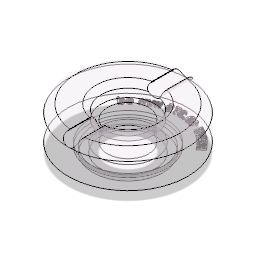
MaxWell_Well_Adapter__Latest_v3 (Autodesk Fusion 360 design; units mm, degrees)
Autodesk Fusion 360 part; units mm, degrees
note: some values were not read from the file. Set by a fixed rule: which face or edge a step refers to.
sketch "Sketch1" plane through (0, 0, 0) normal (0, 1, 0) x (1, 0, 0)
  circle A0 centre (0, 0) radius 16.5
  circle A1 centre (0, 0) radius 5.692
  circle A2 centre (0, 0) radius 7.367
  dimension "d2" = 33
  dimension "d7" = 11.384
  dimension "d21" = 14.734
  constraint coincident A0.centre A1.centre
  constraint concentric A0 A2
  measures "d2" diameter of A0
  measures "d7" diameter of A1
  measures "d21" diameter of A2
extrude "Extrude1" add sketch "Sketch1" along normal blind 9 contours A0
sketch "Sketch2" plane through (0, 0, 0) normal (1, 0, 0) x (0, 0, -1)
  line L0 (16.5, 9) -> (-16.5, 9)
  line L1 (16.5, 0) -> (-16.5, 0)
sketch "Sketch3" plane through (0, 9, 0) normal (0, 1, 0) x (-1, 0, 0)
  circle A0 centre (0, 0) radius 16.5
  line L0 (0, -16.5) -> (0, 16.5)
  line L1 (0, -16.5) -> (0, 16.5)
  line L2 (0, 16.5) -> (-2, 16.5)
  line L3 (0, -16.5) -> (-2, -16.5)
  line L4 (-2, -16.5) -> (-2, 16.5)
  line L5 (-2, 16.5) -> (0, 16.5)
  line L6 (0, 16.5) -> (0, -16.5)
  circle A1 centre (0, 0) radius 7.367
  dimension "d8" = 2
  constraint coincident L0.start L1.start
  constraint coincident L0.end L1.end
  constraint perpendicular L1 L2
  constraint horizontal L3
  constraint vertical L4
  constraint horizontal L5
  constraint vertical L6
  measures "d8" distance of L0.end L2.end
extrude "Extrude3" add sketch "Sketch1" along normal blind 5.95 contours A2
revolve "Revolve1" cut sketch "Sketch3" angle 360 about axis through (0, 9, 16.5) along (0, 0, -1) contours A0 L0 L1 L4 L6 A1 | A0 L2 L4 L5 | A0 L3 L4 | A0 L0 L1 L4 L6 A1 | L0 L1 L4 L6 A1
extrude "Extrude2" add 2 faces at (-4.3141, 9, -12.7105) (4.3141, 9, -12.7105) along direction (0, 1, 0) blind 0.2
fillet "Fillet2" radius 2.2 2 edges at (-16.5, 9.2, 0) (16.5, 9.2, 0)
fillet "Fillet3" radius 1.5 2 edges at (7.367, 9.2, 0) (-7.367, 9.2, 0)
sketch "Sketch5" plane through (0, 0, 0) normal (0, -1, 0) x (1, 0, 0)
  circle A0 centre (0, 0) radius 5.692
  circle A1 centre (0, 0) radius 16.5
  circle A2 centre (0, 0) radius 10.6875
  circle A3 centre (0, 0) radius 9.6875
  circle A4 centre (0, 0) radius 7.6875
  dimension "d29" = 21.375
  dimension "d30" = 19.375
  dimension "d32" = -2
  constraint concentric A0 A2
  constraint concentric A2 A3
  measures "d29" diameter of A2
  measures "d30" diameter of A3
extrude "Extrude5" add sketch "Sketch5" along normal blind 1 contours A2
extrude "Extrude6" add sketch "Sketch5" along normal blind 2.5 contours A3
sketch "Sketch4" plane through (0, 0, 0) normal (0, -1, 0) x (1, 0, 0)
  circle A0 centre (0, 0) radius 16.5
  arc A1 (-16.5, 0) -> (16.5, 0) centre (0, 0) ccw
  arc A2 (-15.5, 0) -> (15.5, 0) centre (0, 0) ccw
  circle A3 centre (0, 0) radius 10.6875
  dimension "d16" = -1
  dimension "d17" = 2
  text T0 "REV7 19.375 mm od" font "Arial" height 2 bold align centre spacing 1.1 along the path A2 letters at x, y, angle (12.9192, -9.5421, -130.0508) (11.4577, -11.2485, -137.7989) (9.8996, -12.6414, -145.2645) (8.1733, -13.8109, -152.1577) (6.6105, -14.6079, -157.0388) (5.7132, -14.9967, -161.9199) (4.0281, -15.5344, -168.2383) (2.3057, -15.8674, -173.1194) (1.3358, -15.9925, -178.0005) (-0.4324, -16.0423, 175.6812) (-2.1952, -15.8973, 169.3628) (-3.9146, -15.5488, 164.4818) (-4.8848, -15.3173, 157.881) (-7.4101, -14.2679, 148.1233) (-9.6697, -12.7901, 141.5226) (-10.4449, -12.189, 136.3591) (-11.8304, -10.8494, 129.4759)
  constraint coincident A0 A1.start
  constraint coincident A0 A1.end
  constraint coincident A0.centre A1.centre
extrude "Extrude4" add sketch "Sketch4" along normal blind 0.5 text T0
move_face "OffsetFaces1" offset -0.5 1 faces at (-6.7755, 5.95, 0)
equation "puck_od = 33 mm"
equation "d2 = puck_od"
equation "puck_height = 9 mm"
equation "d4 = puck_height"
equation "puck_hole = 11.384 mm"
equation "d7 = puck_hole"
equation "lid_hole_diam = 14.734 mm"
equation "d21 = lid_hole_diam"
equation "d22 = puck_height - lid_hole_depth"
equation "lid_hole_depth = 3.05 mm"
equation "d30 = od"
equation "od = 19.375 mm"
